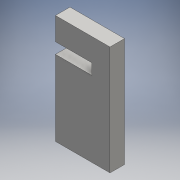
# Autodesk Inventor part: GripperLeftContact
Saved by Autodesk Inventor 2016 (Build 200138000, 138)
## iProperties
Created: 2016-03-31
Part Number: GripperLeftContact
Material: Generic
Document SubType Name: Modeling
Designer: mkepler
Density: 1 g/cm^3
Appearance: Default
Mass: 1.68 g
Surface Area: 12.8 cm^2
Volume: 1.68 cm^3
Author: mkepler
Autodesk Inventor part; units mm, degrees
ref_plane "YZ Plane" through (0, 0, 0) normal (1, 0, 0) x (0, 1, 0)
ref_plane "XZ Plane" through (0, 0, 0) normal (0, 1, 0) x (-1, 0, 0)
ref_plane "XY Plane" through (0, 0, 0) normal (0, 0, 1) x (1, 0, 0)
sketch "Sketch1" plane through (0, 0, 0) normal (0, 1, 0) x (-1, 0, 0)
  line L0 (0, 0) -> (15, 0)
  line L1 (15, -30) -> (0, -30)
  line L2 (0, -30) -> (0, 0)
  line L3 (15, -9.25) -> (5, -9.25)
  line L4 (5, -9.25) -> (5, -6.25)
  line L5 (5, -6.25) -> (15, -6.25)
  line L6 (15, 0) -> (15, -6.25)
  line L7 (15, -9.25) -> (15, -30)
  dimension "d0" = 15
  dimension "d1" = 30
  dimension "d2" = 10
  dimension "d3" = 20.75
  dimension "d6" = 3
  constraints: 16 end point, 5 perpendicular, 3 parallel, 2 horizontal
  measures "d0" distance of L1.start L1.end
  measures "d1" distance of L0.end L1.start
  measures "d2" distance of L3.start L3.end
  measures "d3" distance between parallel lines of L1 L3
  measures "d6" distance between parallel lines of L5 L3
extrude "Extrusion1" add sketch "Sketch1" along normal blind 4
body "Solid1"
